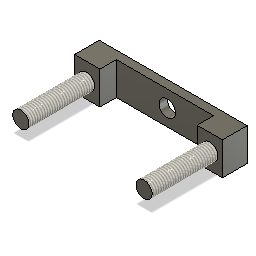
PL_Gripper (Autodesk Fusion 360 design; units mm, degrees)
Autodesk Fusion 360 part; units mm, degrees
note: some values were not read from the file. Set by a fixed rule: which face or edge a step refers to.
sketch "Sketch1" plane through (0, 0, 0) normal (0, 1, 0) x (1, 0, 0)
  line L0 (0, 0) -> (90, 0)
  line L1 (90, 0) -> (90, -5)
  line L2 (90, -5) -> (0, -5)
  line L3 (0, -5) -> (0, 0)
  dimension "d1" = 90
  dimension "d2" = 5
  constraint horizontal L0
  constraint vertical L1
  constraint horizontal L2
  constraint vertical L3
  constraint coincident L0.start L3.end
  measures "d1" distance of L0.start L0.end
  measures "d2" distance of L0.start L2.end
extrude "Extrude1" add sketch "Sketch1" along normal blind 10
extrude "Extrude2" add 1 faces at (30, 10, 1.6667) along direction (0, 1, 0) blind 5
extrude "Extrude3" add 1 faces at (30, 15, 1.6667) along direction (0, 1, 0) blind 5
sketch "Sketch2" plane through (0, 0, 5) normal (0, 0, 1) x (1, 0, 0)
  line L0 (0, 0) -> (90, 0)
  line L1 (90, 0) -> (90, 20)
  line L2 (90, 20) -> (0, 20)
  line L3 (0, 20) -> (0, 0)
  line L4 (0, 0) -> (15.42, 0)
  line L5 (15.42, 20) -> (0, 20)
  line L6 (15.42, 20) -> (15.42, 0)
  line L7 (0, 0) -> (0, 20)
  line L8 (90, 0) -> (74.58, 0)
  line L9 (74.58, 0) -> (74.58, 20)
  line L10 (74.58, 20) -> (90, 20)
  line L11 (90, 0) -> (90, 20)
  dimension "d9" = 15.42
  dimension "d10" = 15.42
  constraint coincident L0.start L3.end
  constraint coincident L0 L4.end
  constraint coincident L2 L5.start
  constraint coincident L2.end L3.start
  constraint perpendicular L3 L5
  constraint perpendicular L4 L6
  constraint coincident L0.end L1.start
  constraint perpendicular L1 L8
  constraint coincident L2 L9.end
  constraint perpendicular L2 L9
  constraint coincident L1.end L2.start
  measures "d9" distance of L0.start L4.end
  measures "d10" distance of L0.end L8.end
extrude "Extrude4" add sketch "Sketch2" along normal blind 10 contours L0 L2 L3 L4 L5 L6 L7 | L0 L1 L2 L8 L9 L10 L11
sketch "Sketch3" plane through (0, 0, 15) normal (0, 0, 1) x (1, 0, 0)
  line L0 (15.42, 20) -> (0, 20)
  line L1 (0, 20) -> (0, 0)
  line L2 (0, 0) -> (15.42, 0)
  line L3 (15.42, 0) -> (15.42, 20)
  circle A0 centre (7.2922, 9.4249) radius 5
  dimension "d13" = 10
  measures "d13" diameter of A0
sketch "Sketch4" plane through (0, 0, 15) normal (0, 0, 1) x (1, 0, 0)
  line L0 (74.58, 0) -> (90, 0)
  line L1 (90, 0) -> (90, 20)
  line L2 (90, 20) -> (74.58, 20)
  line L3 (74.58, 20) -> (74.58, 0)
  circle A0 centre (82.29, 10.052) radius 5
  dimension "d14" = 10
  measures "d14" diameter of A0
extrude "Extrude5" add sketch "Sketch3" sketch "Sketch4" along normal blind 40 contours A0 of sketch 2 contours A0
thread "Thread1" "ISO Metric profile 10.0 M10x1.5 6g" major diameter 9.85 minor diameter 8.141 pitch 1.5 angle 60 resizes the face on face at (12.286, 9.1757, 41.6667)
thread "Thread2" "ISO Metric profile 10.0 M10x1.5 6g" major diameter 9.85 minor diameter 8.141 pitch 1.5 angle 60 resizes the face on face at (87.2838, 10.3013, 28.3333)
hole "Hole1" at (46.3648, 9.7949, 5) direction (0, 0, -1) diameter 10 depth 20 tip angle 118
